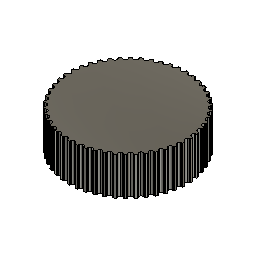
gear_50z (Autodesk Fusion 360 design; units mm, degrees)
Autodesk Fusion 360 part; units mm, degrees
sketch "Sketch1" plane through (0, 0, 0) normal (0, 0, 1) x (1, 0, 0) in component "gt2 pulley"
  circle A0 centre (0, 0) radius 15.9155 construction
  circle A1 centre (0, 0) radius 14.9115 construction
  line L0 (0, 0) -> (0, 15.9155) construction
  line L1 (0, 0) -> (0.9993, 15.8841) construction
  line L2 (0, 0) -> (1.4072, 15.8532) construction
  circle A2 centre (0, 0) radius 15.6615 construction
  arc A3 (0.3879, 15.5215) -> (0.4553, 15.2312) centre (1.3848, 15.6002) ccw
  circle A4 centre (0, 0) radius 15.5115 construction
  arc A5 (0.2406, 15.6596) -> (0, 15.6615) centre (0, 0) ccw
  arc A6 (0.3879, 15.5215) -> (0.2406, 15.6596) centre (0.2383, 15.5097) ccw
  arc A7 (0.4553, 15.2312) -> (0.9363, 14.8821) centre (0.9711, 15.436) ccw
  arc A8 (0, 15.6615) -> (-0.2406, 15.6596) centre (0, 0) ccw
  arc A9 (-0.2406, 15.6596) -> (-0.3879, 15.5215) centre (-0.2383, 15.5097) ccw
  arc A10 (-0.4553, 15.2312) -> (-0.3879, 15.5215) centre (-1.3848, 15.6002) ccw
  arc A11 (-0.9363, 14.8821) -> (-0.4553, 15.2312) centre (-0.9711, 15.436) ccw
  arc A12 (0.9363, 14.8821) -> (-0.9363, 14.8821) centre (0, 0) ccw
  point P0 (1.3848, 15.6002)
  point P1 (0, 15.6615)
  dimension "d18" = 31.831
  dimension "d19" = 3.6
  dimension "d22" = 1.004
  dimension "d24" = 0.75
  dimension "d26" = 1
  dimension "d27" = 0.15
  dimension "d28" = 0.15
  dimension "d47" = 0.555
  dimension "d52" = 3.812
  constraint coincident A0.centre A1.centre
  constraint coincident A0 L0.end
  constraint vertical L0
  constraint coincident A0 L1.end
  constraint coincident A0 L2.end
  constraint concentric A1 A2
  constraint coincident A1 A7.end
  constraint coincident L1 A7.end
  constraint coincident A2 P0
  constraint coincident L2 P0
  constraint coincident P0 A3.centre
  constraint coincident A2 P1
  constraint coincident L0 P1
  constraint concentric A2 A4
  constraint coincident P1 A5.end
  constraint coincident A4 A6.centre
  constraint coincident A3.start A6.start
  constraint tangent A3 A6
  constraint tangent A3 A7
  constraint symmetric L0 A7.end A11.start
  constraint symmetric L0 A3.start A9.end
  constraint symmetric L0 A3.end A10.start
  constraint symmetric L0 A3 A10
  constraint symmetric L0 A5.start A8.end
  constraint symmetric L0 P1 A5.end
  constraint symmetric L0 A5 A8
  constraint symmetric L0 A6 A9
  constraint symmetric L0 A7 A11
  constraint coincident A1 A11.start
  constraint tangent A1 A7
  constraint coincident L1 A7.centre
  measures "d18" diameter of A0
  measures "d19" angle of L0 L1
  measures "d22" distance of A0 A1
  measures "d24" distance of A1 A2
  measures "d26" radius of A3
  measures "d27" distance of A2 A4
  measures "d28" radius of A6
  measures "d47" radius of A7
extrude "Extrude1" add sketch "Sketch1" along normal blind 10 makes body 1
pattern_circular "C-Pattern1" count 50 over 360 about axis through (0, 0, 1.75) along (0, 0, 1) of bodies 1 makes body 2 at (-1.144, 14.8675, 6.6667) makes body 3 at (-4.2101, 14.3048, 6.6667) makes body 4 at (-4.8055, 14.116, 6.6667) makes body 5 at (-7.6353, 12.8084, 6.6667) makes body 6 at (-8.165, 12.4774, 3.3333) makes body 7 at (-9.822, 11.2196, 3.3333) makes body 8 at (-11.4229, 9.5849, 6.6667) makes body 9 at (-12.6457, 7.9019, 3.3333) makes body 10 at (-13.1661, 7.0005, 6.6667) makes body 11 at (-14.3898, 3.9096, 6.6667) makes body 12 at (-14.4934, 3.5063, 6.6667) makes body 13 at (-14.91, 0.2082, 6.6667) makes body 14 at (-14.8882, -0.8324, 6.6667) makes body 15 at (-14.6665, -2.6918, 6.6667) makes body 16 at (-14.0122, -5.1, 6.6667) makes body 17 at (-13.5363, -6.2547, 6.6667) makes body 18 at (-12.6457, -7.9019, 6.6667) makes body 19 at (-11.9401, -8.9323, 3.3333) makes body 20 at (-10.7264, -10.3584, 6.6667) makes body 21 at (-8.3384, -12.3622, 6.6667) makes body 22 at (-7.2747, -13.0166, 6.6667) makes body 23 at (-5.0021, -14.0475, 6.6667) makes body 24 at (-3.8091, -14.4168, 6.6667) makes body 25 at (-2.5894, -14.685, 6.6667) makes body 26 at (0.5204, -14.9024, 6.6667) makes body 27 at (1.7656, -14.8066, 6.6667) makes body 28 at (4.2101, -14.3048, 6.6667) makes body 29 at (4.8055, -14.116, 6.6667) makes body 30 at (7.6353, -12.8084, 6.6667) makes body 31 at (8.165, -12.4774, 6.6667) makes body 32 at (9.822, -11.2196, 3.3333) makes body 33 at (11.8142, -9.0982, 6.6667) makes body 34 at (12.8614, -7.5457, 6.6667) makes body 35 at (13.1661, -7.0005, 6.6667) makes body 36 at (14.3898, -3.9096, 6.6667) makes body 37 at (14.4934, -3.5063, 6.6667) makes body 38 at (14.91, -0.2082, 6.6667) makes body 39 at (14.8882, 0.8324, 6.6667) makes body 40 at (14.6665, 2.6918, 6.6667) makes body 41 at (14.2135, 4.5088, 6.6667) makes body 42 at (13.5363, 6.2547, 6.6667) makes body 43 at (12.6457, 7.9019, 6.6667) makes body 44 at (11.9401, 8.9323, 6.6667) makes body 45 at (9.6644, 11.3557, 6.6667) makes body 46 at (8.3384, 12.3622, 6.6667) makes body 47 at (7.2747, 13.0166, 6.6667) makes body 48 at (5.0021, 14.0475, 6.6667) makes body 49 at (3.8091, 14.4168, 6.6667) makes body 50 at (2.5894, 14.685, 6.6667)
sketch "Sketch2" plane through (0, 0, 10) normal (0, 0, 1) x (-1, 0, 0)
  arc A0 (-9.4371, -12.3292) -> (-9.3991, -12.5275) centre (-9.3092, -12.4075) ccw
  arc A1 (-9.3991, -12.5275) -> (-9.0099, -12.8103) centre (0, 0) ccw
  arc A2 (-9.0099, -12.8103) -> (-8.8095, -12.7851) centre (-8.9235, -12.6877) ccw
  arc A3 (-8.5843, -12.5899) -> (-8.8095, -12.7851) centre (-8.0493, -13.4347) ccw
  arc A4 (-7.99, -12.5902) -> (-8.5843, -12.5899) centre (-8.2874, -13.0588) ccw
  arc A5 (-9.5049, -11.4895) -> (-7.99, -12.5902) centre (0, 0) ccw
  arc A6 (-9.321, -12.0547) -> (-9.5049, -11.4895) centre (-9.8587, -11.9171) ccw
  arc A7 (-9.4371, -12.3292) -> (-9.321, -12.0547) centre (-10.2898, -11.8069) ccw
  circle A8 centre (0, 0) radius 14.9115
  constraint coincident A1.centre A5.centre
extrude "Extrude2" add sketch "Sketch2" against normal blind 10 contours A5 A8 bodies 1 2 3 4 5 6 7 8 9 10 11 12 13 14 15 16 17 18 19 20 21 22 23 24 25 26 27 28 29 30 31 32 33 34 35 36 37 38 39 40 41 42 43 44 45 46 47 48 49 50
extrude "Extrude4" [suppressed] in component "gt2 pulley"
pattern_circular "C-Pattern7" [suppressed] in component "gt2 pulley"
extrude "Extrude3" [suppressed] in component "gt2 pulley"
pattern_circular "C-Pattern6" [suppressed] in component "gt2 pulley"
extrude "Extrude2'" [suppressed] in component "gt2 pulley"
pattern_circular "C-Pattern5" [suppressed] in component "gt2 pulley"
extrude "Extrude1'" [suppressed] in component "gt2 pulley"
pattern_circular "C-Pattern4" [suppressed] in component "gt2 pulley"
pattern_circular "C-Pattern3" [suppressed] in component "gt2 pulley"
pattern_circular "C-Pattern2" [suppressed] in component "gt2 pulley"
pattern_circular "C-Pattern1'" [suppressed] in component "gt2 pulley"
copy_body "Body->Comp1" [suppressed] in component "Component"
copy_body "Body->Comp2" [suppressed] in component "Component'"
copy_body "Body->Comp3" [suppressed] in component "Component''"
copy_body "Body->Comp4" [suppressed] in component "Component'''"
copy_body "Body->Comp5" [suppressed] in component "Component''''"
copy_body "Body->Comp6" [suppressed] in component "Component'''''"
copy_body "Body->Comp7" [suppressed] in component "Component''''''"
copy_body "Body->Comp8" [suppressed] in component "Component'''''''"
copy_body "Body->Comp9" [suppressed] in component "Component''''''''"
copy_body "Body->Comp10" [suppressed] in component "Component'''''''''"
copy_body "Body->Comp11" [suppressed] in component "Component''''''''''"
copy_body "Body->Comp12" [suppressed] in component "Component'''''''''''"
copy_body "Body->Comp13" [suppressed] in component "Component''''''''''''"
copy_body "Body->Comp14" [suppressed] in component "Component'''''''''''''"
copy_body "Body->Comp15" [suppressed] in component "Component''''''''''''''"
copy_body "Body->Comp16" [suppressed] in component "Component'''''''''''''''"
copy_body "Body->Comp17" [suppressed] in component "Component''''''''''''''''"
copy_body "Body->Comp18" [suppressed] in component "Component'''''''''''''''''"
copy_body "Body->Comp19" [suppressed] in component "Component''''''''''''''''''"
copy_body "Body->Comp20" [suppressed] in component "Component'''''''''''''''''''"
component "gt2 pulley" placed x (1, 0, 0) y (0, 1, 0) z (0, 0, 1) at (0, 0, 0)
equation "NumTeeth = 50" comment "min 20"
equation "ToothPitch = 2 mm"
equation "PullyDia = NumTeeth * ToothPitch / PI"
equation "ToothAng = ( ( 360 / NumTeeth ) * 1 deg )"
equation "TransOffsetAngle = ToothAng * 0.2"
equation "Sholulder_Radius = 0.15 mm"
equation "Root_Radius = 0.555 mm"
equation "TransRadius = 1 mm"
equation "ToolHeight = 0.75 mm"
equation "PLD = 0.254 mm"
equation "d18 = PullyDia"
equation "d19 = ToothAng / 2"
equation "d22 = PLD + ToolHeight"
equation "d24 = ToolHeight"
equation "d26 = TransRadius"
equation "d27 = Sholulder_Radius"
equation "d31 = NumTeeth"
equation "d33 = NumTeeth"
equation "d35 = NumTeeth"
equation "d37 = NumTeeth"
equation "d41 = NumTeeth"
equation "d45 = NumTeeth"
equation "d47 = Root_Radius"
equation "d50 = NumTeeth"
